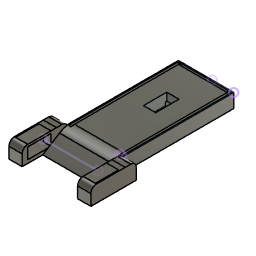
BottomPlate (Autodesk Fusion 360 design; units mm, degrees)
Autodesk Fusion 360 part; units mm, degrees
sketch "Sketch1" plane through (0, 0, 0) normal (0, 0, 1) x (1, 0, 0)
  line L0 (0, 0) -> (50, 0)
  line L1 (50, 0) -> (50, -122.5)
  line L2 (50, -122.5) -> (0, -122.5)
  line L3 (0, -122.5) -> (0, 0)
  dimension "d1" = 50
  dimension "d2" = 122.5
  constraint horizontal L0
  constraint vertical L1
  constraint horizontal L2
  constraint vertical L3
  constraint coincident L0.start L3.end
  measures "d1" distance of L0.start L0.end
  measures "d2" distance of L0.start L2.end
extrude "Extrude1" add sketch "Sketch1" along normal blind 15
sketch "Sketch2" plane through (50, 0, 0) normal (1, 0, 0) x (0, 1, 0)
  line L0 (-122.5, 0) -> (0, 0)
  line L1 (0, 0) -> (0, 15)
  line L2 (0, 15) -> (-122.5, 15)
  line L3 (-122.5, 15) -> (-122.5, 0)
  line L4 (-102.5, 15) -> (-122.5, 0)
  line L5 (-102.5, 15) -> (-122.5, 15)
  line L6 (-122.5, 0) -> (-122.5, 15)
  constraint coincident L0.start L3.end
  constraint coincident L2 L4.start
  constraint coincident L2.end L3.start
  constraint perpendicular L3 L5
sketch "Sketch3" plane through (50, 0, 0) normal (1, 0, 0) x (0, 1, 0)
extrude "Extrude2" cut sketch "Sketch2" against normal blind 67 contours L2 L3 L4 L5 L6
sketch "Sketch4" plane through (0, 0, 15) normal (0, 0, 1) x (-1, 0, 0)
  line L0 (0, 102.5) -> (-50, 102.5)
  line L1 (-50, 102.5) -> (-50, 0)
  line L2 (-50, 0) -> (0, 0)
  line L3 (0, 0) -> (0, 102.5)
  line L4 (-25, 30) -> (-30.5, 30)
  line L5 (-25, 30) -> (-19.5, 30)
  line L6 (-19.5, 30) -> (-30.5, 30)
  line L7 (-30.5, 30) -> (-30.5, 51)
  line L8 (-30.5, 51) -> (-19.5, 51)
  line L9 (-19.5, 51) -> (-19.5, 30)
  dimension "d8" = 5.5
  dimension "d9" = 5.5
  dimension "d10" = 11
  dimension "d11" = 21
  constraint parallel L4 L5
  constraint horizontal L6
  constraint vertical L7
  constraint horizontal L8
  constraint vertical L9
  measures "d8" distance of L4.start L4.end
  measures "d9" distance of L4.start L5.end
  measures "d10" distance of L5.end L4.end
  measures "d11" distance of L5.end L8.end
extrude "Extrude3" cut sketch "Sketch4" against normal blind 10 contours L4 L5 L6 L7 L8 L9
sketch "Sketch5" plane through (0, 0, 5) normal (0, 0, 1) x (-1, 0, 0)
  line L0 (-19.5, 51) -> (-30.5, 51)
  line L1 (-30.5, 51) -> (-30.5, 30)
  line L2 (-30.5, 30) -> (-19.5, 30)
  line L3 (-19.5, 30) -> (-19.5, 51)
extrude "Extrude4" add sketch "Sketch2" against normal up to surface (50 mm away) contours L2 L3 L4 L5 L6
sketch "Sketch6" plane through (19.5, 0, 0) normal (1, 0, 0) x (0, 1, 0)
  line L0 (-30, 15) -> (-51, 15)
  line L1 (-51, 15) -> (-51, 5)
  line L2 (-51, 5) -> (-30, 5)
  line L3 (-30, 5) -> (-30, 15)
extrude "Extrude5" cut 1 faces at (16.6667, -40.8333, 0) along direction (0, 0, 1) blind 2.5
sketch "Sketch7" plane through (50, 0, 0) normal (1, 0, 0) x (0, 1, 0)
  line L0 (-122.5, 2.5) -> (0, 2.5)
  line L1 (0, 2.5) -> (0, 15)
  line L2 (0, 15) -> (-122.5, 15)
  line L3 (-122.5, 15) -> (-122.5, 2.5)
  line L4 (-102.5, 15) -> (-122.5, 2.5)
  line L5 (-122.5, 2.5) -> (-122.5, 15)
  line L6 (-102.5, 15) -> (-122.5, 15)
  constraint coincident L2 L4.start
  constraint coincident L0.start L3.end
  constraint coincident L2.end L3.start
  constraint perpendicular L5 L6
extrude "Extrude6" cut sketch "Sketch7" against normal blind 51 contours L2 L3 L4 L5 L6
sketch "Sketch8" plane through (0, 0, 5) normal (0, 0, 1) x (-1, 0, 0)
  line L0 (-30.465, 31.0492) -> (-19.4899, 31.0492)
  line L1 (-19.4899, 31.0492) -> (-19.4899, -8.9508)
  line L2 (-19.4899, -8.9508) -> (-30.465, -8.9508)
  line L3 (-30.465, -8.9508) -> (-30.465, 31.0492)
  dimension "d21" = 40
  constraint horizontal L0
  constraint vertical L1
  constraint horizontal L2
  constraint vertical L3
  measures "d21" distance of L0 L2
extrude "Extrude7" cut sketch "Sketch8" along normal blind 3 and the other way blind 7
sketch "Sketch9" plane through (0, 0, 15) normal (0, 0, 1) x (-1, 0, 0)
  line L0 (0, 102.5) -> (-50, 102.5)
  line L1 (-50, 102.5) -> (-50, 0)
  line L2 (-50, 0) -> (0, 0)
  line L3 (0, 0) -> (0, 102.5)
  line L4 (-30.5, 30) -> (-30.5, 51)
  line L5 (-30.5, 51) -> (-19.5, 51)
  line L6 (-19.5, 51) -> (-19.5, 30)
  line L7 (-19.5, 30) -> (-30.5, 30)
  line L8 (0, 0) -> (0, 1)
  line L9 (0, 1) -> (-1, 1)
  line L10 (-1, 1) -> (-3, 1)
  line L11 (-3, 1) -> (-3, 100)
  line L12 (-3, 100) -> (-1, 100)
  line L13 (-1, 100) -> (-1, 1)
  line L14 (-25, 0) -> (-25, 102.5)
  line L15 (-47, 100) -> (-49, 100)
  line L16 (-49, 100) -> (-49, 1)
  line L17 (-47, 1) -> (-47, 100)
  line L18 (-49, 1) -> (-47, 1)
  dimension "d28" = 99
  constraint coincident L2.end L3.start
  constraint coincident L3 L8.end
  constraint perpendicular L3 L9
  constraint horizontal L10
  constraint vertical L11
  constraint horizontal L12
  constraint vertical L13
  constraint midpoint L2 L14.start
  constraint midpoint L0 L14.end
  constraint symmetric L9.end L14 L16.end
  constraint symmetric L10.end L14 L17.start
  constraint symmetric L11.end L14 L15.start
  constraint symmetric L12.end L14 L15.end
  measures "d28" distance of L10.end L11.end
extrude "Extrude8" cut sketch "Sketch9" against normal blind 3 contours L10 L11 L12 L13 | L15 L16 L17 L18
sketch "Sketch10" plane through (0, 0, 15) normal (0, 0, 1) x (-1, 0, 0)
  line L0 (-3, 1) -> (-3, 100)
  line L1 (-3, 100) -> (-1, 100)
  line L2 (-1, 100) -> (-1, 1)
  line L3 (-1, 1) -> (-3, 1)
  line L4 (-47, 100) -> (-47, 1)
  line L5 (-47, 1) -> (-49, 1)
  line L6 (-49, 1) -> (-49, 100)
  line L7 (-49, 100) -> (-47, 100)
  line L8 (0, 102.5) -> (-50, 102.5)
  line L9 (-50, 102.5) -> (-50, 0)
  line L10 (-50, 0) -> (0, 0)
  line L11 (0, 0) -> (0, 102.5)
  line L12 (-30.5, 30) -> (-30.5, 51)
  line L13 (-30.5, 51) -> (-19.5, 51)
  line L14 (-19.5, 51) -> (-19.5, 30)
  line L15 (-19.5, 30) -> (-30.5, 30)
  line L16 (-3.5, 1) -> (-46.5, 1)
  line L17 (-46.5, 1) -> (-46.5, 3)
  line L18 (-46.5, 3) -> (-3.5, 3)
  line L19 (-3.5, 3) -> (-3.5, 1)
  dimension "d31" = 43
  dimension "d32" = 0.5
  constraint horizontal L16
  constraint vertical L17
  constraint horizontal L18
  constraint vertical L19
  measures "d31" distance of L17.end L18.end
  measures "d32" distance of L4 L17
extrude "Extrude9" cut sketch "Sketch10" against normal blind 3 contours L16 L17 L18 L19
sketch "Sketch11" plane through (0, 0, 15) normal (0, 0, 1) x (-1, 0, 0)
  line L0 (-46.5, 1) -> (-46.5, 3)
  line L1 (-46.5, 3) -> (-3.5, 3)
  line L2 (-3.5, 3) -> (-3.5, 1)
  line L3 (-3.5, 1) -> (-46.5, 1)
  line L4 (-3, 1) -> (-3, 100)
  line L5 (-3, 100) -> (-1, 100)
  line L6 (-1, 100) -> (-1, 1)
  line L7 (-1, 1) -> (-3, 1)
  line L8 (-47, 100) -> (-47, 1)
  line L9 (-47, 1) -> (-49, 1)
  line L10 (-49, 1) -> (-49, 100)
  line L11 (-49, 100) -> (-47, 100)
  line L12 (0, 102.5) -> (-50, 102.5)
  line L13 (-50, 102.5) -> (-50, 0)
  line L14 (-50, 0) -> (0, 0)
  line L15 (0, 0) -> (0, 102.5)
  line L16 (-30.5, 30) -> (-30.5, 51)
  line L17 (-30.5, 51) -> (-19.5, 51)
  line L18 (-19.5, 51) -> (-19.5, 30)
  line L19 (-19.5, 30) -> (-30.5, 30)
sketch "Sketch12" plane through (50, 0, 0) normal (1, 0, 0) x (0, 1, 0)
  line L0 (-102.5, 15) -> (-122.5, 2.5)
  line L1 (-122.5, 2.5) -> (0, 2.5)
  line L2 (0, 2.5) -> (0, 15)
  line L3 (0, 15) -> (-102.5, 15)
sketch "Sketch13" plane through (50, 0, 0) normal (1, 0, 0) x (0, 1, 0)
sketch "Sketch14" plane through (50, 0, 0) normal (1, 0, 0) x (0, 1, 0)
  line L0 (-110, 10) -> (-110, 17.5)
  line L1 (-121, 3) -> (-121, 7.5)
  line L2 (-121, 7.5) -> (-141, 7.5)
  line L3 (-141, 7.5) -> (-141, 17.5)
  line L4 (-141, 17.5) -> (-110, 17.5)
  line L5 (-110, 10) -> (-100, 10)
  line L6 (-121, 3) -> (-100, 3)
  line L7 (-100, 3) -> (-100, 10)
  dimension "d33" = 20
  dimension "d34" = 10
  dimension "d35" = 10
  constraint vertical L0
  constraint vertical L1
  constraint perpendicular L1 L2
  constraint perpendicular L2 L3
  constraint perpendicular L3 L4
  constraint perpendicular L0 L5
  constraint perpendicular L1 L6
  constraint parallel L1 L7
  measures "d33" distance of L1.end L2.end
  measures "d34" distance of L2.end L3.end
  measures "d35" distance of L0.start L5.end
extrude "Extrude10" add sketch "Sketch14" along normal blind 12
sketch "Sketch15" plane through (0, 0, 17.5) normal (0, 0, 1) x (-1, 0, 0)
  line L0 (-50, 110) -> (-50, 141)
  line L1 (-50, 141) -> (-62, 141)
  line L2 (-62, 141) -> (-62, 110)
  line L3 (-62, 110) -> (-50, 110)
  line L4 (-50, 136) -> (-61, 136)
  line L5 (-61, 136) -> (-61, 115)
  line L6 (-61, 115) -> (-50, 115)
  line L7 (-50, 115) -> (-50, 136)
  constraint horizontal L4
  constraint vertical L5
  constraint horizontal L6
  constraint vertical L7
  constraint coincident L0 L4.start
extrude "Extrude11" cut sketch "Sketch15" against normal blind 10 contours L0 L4 L5 L6 L7
extrude "Extrude12" add 1 faces at (57.6667, -121, 4.6458) along direction (0, -1, 0) up to surface (20 mm away)
extrude "Extrude13" add 1 faces at (58, -110, 12.6042) along direction (0, 1, 0) up to surface (10 mm away)
sketch "Sketch16" plane through (0, -115, 0) normal (0, -1, 0) x (1, 0, 0)
  line L0 (61, 17.5) -> (50, 17.5)
  line L1 (50, 17.5) -> (50, 7.5)
  line L2 (50, 7.5) -> (61, 7.5)
  line L3 (61, 7.5) -> (61, 17.5)
  line L4 (61, 7.5) -> (56.68, 7.5)
  line L5 (56.68, 7.5) -> (56.68, 17.5)
  line L6 (61, 17.5) -> (61, 7.5)
  constraint horizontal L4
  constraint vertical L5
  constraint vertical L6
  constraint coincident L0 L5.end
  constraint coincident L2.end L3.start
sketch "Sketch17" plane through (0, -115, 0) normal (0, -1, 0) x (1, 0, 0)
  line L0 (61, 17.5) -> (50, 17.5)
  line L1 (50, 17.5) -> (50, 7.5)
  line L2 (50, 7.5) -> (61, 7.5)
  line L3 (61, 7.5) -> (61, 17.5)
extrude "Extrude14" cut 1 faces at (53.6667, -122, 7.5) along direction (0, 0, -1) blind 2
sketch "Sketch18" plane through (50, 0, 0) normal (-1, 0, 0) x (0, -1, 0)
  line L0 (136, 5.5) -> (117.7, 5.5)
  line L1 (117.7, 5.5) -> (121.7, 3)
  line L2 (121.7, 3) -> (141, 3)
  line L3 (141, 3) -> (141, 17.5)
  line L4 (141, 17.5) -> (136, 17.5)
  line L5 (136, 17.5) -> (136, 5.5)
  line L6 (114.9201, 17.4881) -> (114.9201, 15.4881)
  line L7 (114.9201, 17.4881) -> (136, 17.4881)
  line L8 (136, 17.4881) -> (136, 15.4881)
  line L9 (136, 15.4881) -> (114.9201, 15.4881)
  line L10 (114.9201, 15.4881) -> (114.9201, 17.4881)
  dimension "d48" = 2
  constraint vertical L6
  constraint horizontal L7
  constraint vertical L8
  constraint horizontal L9
  constraint vertical L10
  constraint coincident L5 L8.end
  measures "d48" distance of L6.start L6.end
extrude "Extrude15" add sketch "Sketch18" against normal blind 12 contours L5 L6 L7 L8 L9 L10
sketch "Sketch19" plane through (0, -115, 0) normal (0, -1, 0) x (1, 0, 0)
  line L0 (61, 15.4881) -> (50, 15.4881)
  line L1 (50, 15.4881) -> (50, 7.1875)
  line L2 (50, 7.1875) -> (50, 5.5)
  line L3 (50, 5.5) -> (61, 5.5)
  line L4 (61, 5.5) -> (61, 15.4881)
  line L5 (61, 5.5) -> (56.9549, 5.5)
  line L6 (56.9549, 5.5) -> (56.9549, 15.4881)
  line L7 (56.9549, 15.4881) -> (61, 15.4881)
  line L8 (61, 15.4881) -> (61, 5.5)
  constraint horizontal L5
  constraint vertical L6
  constraint horizontal L7
  constraint vertical L8
  constraint coincident L0 L6.end
  constraint coincident L3.end L4.start
extrude "Extrude16" cut sketch "Sketch19" against normal blind 22 contours L0 L3 L4 L5 L6 L7 L8
sketch "Sketch20" plane through (50, 0, 0) normal (-1, 0, 0) x (0, -1, 0)
  line L0 (136, 5.5) -> (117.7, 5.5)
  line L1 (117.7, 5.5) -> (121.7, 3)
  line L2 (121.7, 3) -> (141, 3)
  line L3 (141, 3) -> (141, 17.5)
  line L4 (141, 17.5) -> (136, 17.5)
  line L5 (136, 17.5) -> (136, 17.4881)
  line L6 (136, 17.4881) -> (115, 17.4881)
  line L7 (115, 17.4881) -> (115, 17.5)
  line L8 (115, 17.5) -> (110, 17.5)
  line L9 (110, 17.5) -> (100, 17.5)
  line L10 (100, 17.5) -> (100, 15)
  line L11 (100, 15) -> (102.5, 15)
  line L12 (102.5, 15) -> (115, 7.1875)
  line L13 (115, 7.1875) -> (115, 15.4881)
  line L14 (115, 15.4881) -> (136, 15.4881)
  line L15 (136, 15.4881) -> (136, 5.5)
sketch "Sketch21" plane through (0, 0, 15) normal (0, 0, 1) x (-1, 0, 0)
  line L0 (-46.5, 1) -> (-46.5, 3)
  line L1 (-46.5, 3) -> (-3.5, 3)
  line L2 (-3.5, 3) -> (-3.5, 1)
  line L3 (-3.5, 1) -> (-46.5, 1)
  line L4 (-3, 1) -> (-3, 100)
  line L5 (-3, 100) -> (-1, 100)
  line L6 (-1, 100) -> (-1, 1)
  line L7 (-1, 1) -> (-3, 1)
  line L8 (-47, 100) -> (-47, 1)
  line L9 (-47, 1) -> (-49, 1)
  line L10 (-49, 1) -> (-49, 100)
  line L11 (-49, 100) -> (-47, 100)
  line L12 (0, 102.5) -> (-50, 102.5)
  line L13 (-50, 102.5) -> (-50, 100)
  line L14 (-50, 100) -> (-50, 0)
  line L15 (-50, 0) -> (0, 0)
  line L16 (0, 0) -> (0, 102.5)
  line L17 (-30.5, 30) -> (-30.5, 51)
  line L18 (-30.5, 51) -> (-19.5, 51)
  line L19 (-19.5, 51) -> (-19.5, 30)
  line L20 (-19.5, 30) -> (-30.5, 30)
  line L21 (0, 102.5) -> (-50, 102.5)
  line L22 (-25, 102.5) -> (-25, 139)
  constraint coincident L12.start L16.end
  constraint coincident L12.end L13.start
  constraint midpoint L21 L22.start
  constraint perpendicular L21 L22
ref_plane "WorkPlane1" through (25, -120.5, 10.25) normal (-1, 0, 0) x (0, -1, 0)
mirror "Mirror1" about plane through (25, -120.5, 10.25) normal (-1, 0, 0) of "Extrude10", "Extrude11", "Extrude12", "Extrude13", "Extrude14", "Extrude15", "Extrude16"
fillet "Fillet1" radius 5 1 edges at (56, -100, 17.5)
fillet "Fillet2" radius 5 1 edges at (-6, -100, 17.5)
fillet "Fillet3" radius 20 1 edges at (25, -102.5, 15)
fillet "Fillet4" radius 5 1 edges at (-6, -141, 17.5)
fillet "Fillet5" radius 5 1 edges at (56, -141, 17.5)
extrude "Extrude17" add 2 faces at (-8, -120.9, 3) (58, -120.9, 3) along direction (0, 0, -1) up to surface end surface through (0, 0, 2.5) normal (0, 0, -1) offset 0
sketch "Sketch22" plane through (0, 0, 15) normal (0, 0, 1) x (-1, 0, 0)
  line L0 (-30.5, 30) -> (-30.5, 51)
  line L1 (-30.5, 51) -> (-19.5, 51)
  line L2 (-19.5, 51) -> (-19.5, 30)
  line L3 (-19.5, 30) -> (-30.5, 30)
  line L4 (0, 96.7641) -> (-1, 96.7641)
  line L5 (-1, 96.7641) -> (-1, 1)
  line L6 (-1, 1) -> (-3, 1)
  line L7 (-3, 1) -> (-3, 96.7641)
  line L8 (-3, 96.7641) -> (-47, 96.7641)
  line L9 (-47, 96.7641) -> (-47, 1)
  line L10 (-47, 1) -> (-49, 1)
  line L11 (-49, 1) -> (-49, 96.7641)
  line L12 (-49, 96.7641) -> (-50, 96.7641)
  line L13 (-50, 96.7641) -> (-50, 0)
  line L14 (-50, 0) -> (0, 0)
  line L15 (0, 0) -> (0, 96.7641)
  line L16 (-46.5, 1) -> (-46.5, 3)
  line L17 (-46.5, 3) -> (-3.5, 3)
  line L18 (-3.5, 3) -> (-3.5, 1)
  line L19 (-3.5, 1) -> (-46.5, 1)
  line L20 (0, 122.5) -> (-50, 122.5)
  line L21 (-50, 0) -> (-30.465, 0)
  line L22 (-49, 100) -> (-47, 100)
  point P0 (-50, 0)
  dimension "d70" = 50
  dimension "d72" = 100
  measures "d70" distance of P0 L14.end
  measures "d72" distance of P0 L22
